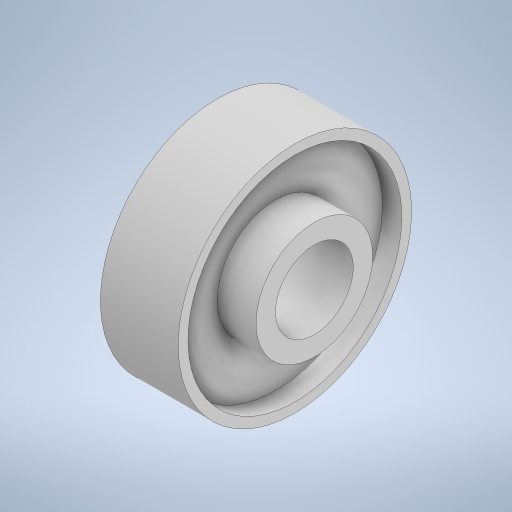
# Autodesk Inventor part: Rueda polea
Saved by Autodesk Inventor 2024 (Build 280153000, 153)
## iProperties
Created: 2024-03-03
Part Number: Rueda polea
Material: Genérico
Document SubType Name: Modeling
Designer: kelly
Density: 1 g/cm^3
Appearance: Valor por defecto
Author: kelly
Autodesk Inventor part; units mm, degrees
ref_plane "YZ Plane" through (0, 0, 0) normal (1, 0, 0) x (0, 1, 0)
ref_plane "XZ Plane" through (0, 0, 0) normal (0, 1, 0) x (-1, 0, 0)
ref_plane "XY Plane" through (0, 0, 0) normal (0, 0, 1) x (1, 0, 0)
sketch "Boceto1" plane through (0, 0, 0) normal (0, 0, 1) x (1, 0, 0)
  line L0 (-15, 0) -> (15, 0)
  line L1 (15, 0) -> (15, 5)
  line L2 (15, 5) -> (5, 5)
  line L3 (5, 5) -> (5, 17.5)
  line L4 (5, 17.5) -> (10, 17.5)
  line L5 (10, 17.5) -> (10, 20)
  line L6 (10, 20) -> (-10, 20)
  line L7 (-10, 20) -> (-10, 17.5)
  line L8 (-10, 17.5) -> (-5, 17.5)
  line L9 (-5, 17.5) -> (-5, 5)
  line L10 (-5, 5) -> (-15, 5)
  line L11 (-15, 5) -> (-15, 0)
  line L12 (-15, -10) -> (15, -10)
  point P0 (0, 0)
  point P1 (0, 0)
  point P2 (7.5, 17.5)
  point P3 (10, 5)
  dimension "d6" = 30
  dimension "d7" = 20
  dimension "d8" = 5
  dimension "d9" = 60
  dimension "d10" = 55
  dimension "d11" = 30
  dimension "d12" = 20
  constraints: 26 end point, 9 perpendicular, 4 point on line, 3 midpoint, 2 collinear, 2 horizontal, 1 coincident
  measures "d6" distance of L0.start L0.end
  measures "d7" distance of L5.end L6.end
  measures "d8" distance of L3.end L4.end
  measures "d9" diameter of L6 L12
  measures "d10" diameter of point (7.5, 17.5) L12
  measures "d11" diameter of point (10, 5) L12
  measures "d12" diameter of L0 L12
revolve "Revolución1" add sketch "Boceto1" angle 360 about axis through (-15, -10, 0) along (1, 0, 0)
